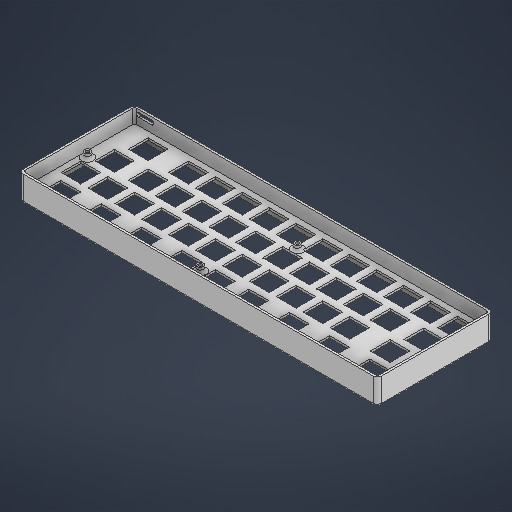
# Autodesk Inventor part: Top
Saved by Autodesk Inventor 2026 (Build 300175050, 175E)
## iProperties
Created: 2025-06-14
Part Number: Top
Material: Generisch
Document SubType Name: Modeling
Designer: nikla
Density: 1 g/cm^3
Appearance: Vorgabe
Author: nikla
Autodesk Inventor part; units mm, degrees
ref_plane "YZ Plane" through (0, 0, 0) normal (1, 0, 0) x (0, 1, 0)
ref_plane "XZ Plane" through (0, 0, 0) normal (0, 1, 0) x (-1, 0, 0)
ref_plane "XY Plane" through (0, 0, 0) normal (0, 0, 1) x (1, 0, 0)
sketch "Skizze1" plane through (0, 0, 0) normal (0, 0, 1) x (1, 0, 0)
  arc A0 (-233.4346, 67.6971) -> (-234.4346, 66.6971) centre (-233.4346, 66.6971) ccw projected
  line L0 (14.5654, 67.6971) -> (-233.4346, 67.6971) projected
  arc A1 (15.5654, 66.6971) -> (14.5654, 67.6971) centre (14.5654, 66.6971) ccw projected
  line L1 (15.5654, -9.3029) -> (15.5654, 66.6971) projected
  arc A2 (14.5654, -10.3029) -> (15.5654, -9.3029) centre (14.5654, -9.3029) ccw projected
  line L2 (-233.4346, -10.3029) -> (14.5654, -10.3029) projected
  arc A3 (-234.4346, -9.3029) -> (-233.4346, -10.3029) centre (-233.4346, -9.3029) ccw projected
  line L3 (-234.4346, 66.6971) -> (-234.4346, -9.3029) projected
  circle A4 centre (11.9054, -6.6429) radius 1.6 projected
  circle A5 centre (5.0729, 0.0071) radius 0.875 projected
  circle A6 centre (-0.0071, 0.0071) radius 2 projected
  circle A7 centre (-5.0871, 0.0071) radius 0.875 projected
  circle A8 centre (-23.5021, 0.0071) radius 0.875 projected
  circle A9 centre (-28.5821, 0.0071) radius 2 projected
  circle A10 centre (-33.6621, 0.0071) radius 0.875 projected
  circle A11 centre (3.8029, 2.5471) radius 0.75 projected
  circle A12 centre (-2.5471, 5.0871) radius 0.75 projected
  circle A13 centre (-24.7721, 2.5471) radius 0.75 projected
  circle A14 centre (-31.1221, 5.0871) radius 0.75 projected
  circle A15 centre (-52.0771, 0.0071) radius 0.875 projected
  circle A16 centre (-57.1571, 0.0071) radius 2 projected
  circle A17 centre (-62.2371, 0.0071) radius 0.875 projected
  circle A18 centre (-80.6521, 0.0071) radius 0.875 projected
  circle A19 centre (-85.7321, 0.0071) radius 2 projected
  circle A20 centre (-90.8121, 0.0071) radius 0.875 projected
  circle A21 centre (-104.4646, 0.0071) radius 0.875 projected
  circle A22 centre (-53.3471, 2.5471) radius 0.75 projected
  circle A23 centre (-59.6971, 5.0871) radius 0.75 projected
  circle A24 centre (-81.9221, 2.5471) radius 0.75 projected
  circle A25 centre (-88.2721, 5.0871) radius 0.75 projected
  circle A26 centre (-105.7346, 2.5471) radius 0.75 projected
  circle A27 centre (0.3104, 19.0571) radius 0.875 projected
  circle A28 centre (-0.9596, 21.5971) radius 0.75 projected
  circle A29 centre (-4.7696, 19.0571) radius 2 projected
  circle A30 centre (-9.8496, 19.0571) radius 0.875 projected
  circle A31 centre (-7.3096, 24.1371) radius 0.75 projected
  circle A32 centre (-28.2646, 19.0571) radius 0.875 projected
  circle A33 centre (-29.5346, 21.5971) radius 0.75 projected
  circle A34 centre (-33.3446, 19.0571) radius 2 projected
  circle A35 centre (-38.4246, 19.0571) radius 0.875 projected
  circle A36 centre (-47.3146, 19.0571) radius 0.875 projected
  circle A37 centre (-35.8846, 24.1371) radius 0.75 projected
  circle A38 centre (-52.3946, 19.0571) radius 2 projected
  circle A39 centre (-57.4746, 19.0571) radius 0.875 projected
  circle A40 centre (-48.5846, 21.5971) radius 0.75 projected
  circle A41 centre (-66.3646, 19.0571) radius 0.875 projected
  circle A42 centre (-71.4446, 19.0571) radius 2 projected
  circle A43 centre (-76.5246, 19.0571) radius 0.875 projected
  circle A44 centre (-67.6346, 21.5971) radius 0.75 projected
  circle A45 centre (-54.9346, 24.1371) radius 0.75 projected
  circle A46 centre (-73.9846, 24.1371) radius 0.75 projected
  circle A47 centre (-85.4146, 19.0571) radius 0.875 projected
  circle A48 centre (-90.4946, 19.0571) radius 2 projected
  circle A49 centre (-86.6846, 21.5971) radius 0.75 projected
  circle A50 centre (-95.5746, 19.0571) radius 0.875 projected
  circle A51 centre (-104.4646, 19.0571) radius 0.875 projected
  circle A52 centre (-105.7346, 21.5971) radius 0.75 projected
  circle A53 centre (-93.0346, 24.1371) radius 0.75 projected
  circle A54 centre (-109.5446, 0.0071) radius 2 projected
  circle A55 centre (-114.6246, 0.0071) radius 0.875 projected
  circle A56 centre (-128.2771, 0.0071) radius 0.875 projected
  circle A57 centre (-133.3571, 0.0071) radius 2 projected
  circle A58 centre (-138.4371, 0.0071) radius 0.875 projected
  circle A59 centre (-156.8521, 0.0071) radius 0.875 projected
  circle A60 centre (-161.9321, 0.0071) radius 2 projected
  circle A61 centre (-167.0121, 0.0071) radius 0.875 projected
  circle A62 centre (-121.1946, 0.9571) radius 1.6 projected
  circle A63 centre (-112.0846, 5.0871) radius 0.75 projected
  circle A64 centre (-129.5471, 2.5471) radius 0.75 projected
  circle A65 centre (-135.8971, 5.0871) radius 0.75 projected
  circle A66 centre (-158.1221, 2.5471) radius 0.75 projected
  circle A67 centre (-164.4721, 5.0871) radius 0.75 projected
  circle A68 centre (-185.4271, 0.0071) radius 0.875 projected
  circle A69 centre (-190.5071, 0.0071) radius 2 projected
  circle A70 centre (-195.5871, 0.0071) radius 0.875 projected
  circle A71 centre (-230.6946, -6.6429) radius 1.6 projected
  circle A72 centre (-214.0021, 0.0071) radius 0.875 projected
  circle A73 centre (-219.0821, 0.0071) radius 2 projected
  circle A74 centre (-224.1621, 0.0071) radius 0.875 projected
  circle A75 centre (-186.6971, 2.5471) radius 0.75 projected
  circle A76 centre (-193.0471, 5.0871) radius 0.75 projected
  circle A77 centre (-215.2721, 2.5471) radius 0.75 projected
  circle A78 centre (-221.6221, 5.0871) radius 0.75 projected
  circle A79 centre (-109.5446, 19.0571) radius 2 projected
  circle A80 centre (-114.6246, 19.0571) radius 0.875 projected
  circle A81 centre (-123.5146, 19.0571) radius 0.875 projected
  circle A82 centre (-128.5946, 19.0571) radius 2 projected
  circle A83 centre (-133.6746, 19.0571) radius 0.875 projected
  circle A84 centre (-124.7846, 21.5971) radius 0.75 projected
  circle A85 centre (-112.0846, 24.1371) radius 0.75 projected
  circle A86 centre (-131.1346, 24.1371) radius 0.75 projected
  circle A87 centre (-142.5646, 19.0571) radius 0.875 projected
  circle A88 centre (-147.6446, 19.0571) radius 2 projected
  circle A89 centre (-152.7246, 19.0571) radius 0.875 projected
  circle A90 centre (-143.8346, 21.5971) radius 0.75 projected
  circle A91 centre (-161.6146, 19.0571) radius 0.875 projected
  circle A92 centre (-166.6946, 19.0571) radius 2 projected
  circle A93 centre (-162.8846, 21.5971) radius 0.75 projected
  circle A94 centre (-150.1846, 24.1371) radius 0.75 projected
  circle A95 centre (-169.2346, 24.1371) radius 0.75 projected
  circle A96 centre (-171.7746, 19.0571) radius 0.875 projected
  circle A97 centre (-180.6646, 19.0571) radius 0.875 projected
  circle A98 centre (-185.7446, 19.0571) radius 2 projected
  circle A99 centre (-181.9346, 21.5971) radius 0.75 projected
  circle A100 centre (-190.8246, 19.0571) radius 0.875 projected
  circle A101 centre (-199.7146, 19.0571) radius 0.875 projected
  circle A102 centre (-200.9846, 21.5971) radius 0.75 projected
  circle A103 centre (-188.2846, 24.1371) radius 0.75 projected
  circle A104 centre (-204.7946, 19.0571) radius 2 projected
  circle A105 centre (-209.8746, 19.0571) radius 0.875 projected
  circle A106 centre (-218.7646, 19.0571) radius 0.875 projected
  circle A107 centre (-223.8446, 19.0571) radius 2 projected
  circle A108 centre (-228.9246, 19.0571) radius 0.875 projected
  circle A109 centre (-220.0346, 21.5971) radius 0.75 projected
  circle A110 centre (-207.3346, 24.1371) radius 0.75 projected
  circle A111 centre (-226.3846, 24.1371) radius 0.75 projected
  circle A112 centre (5.0729, 38.1071) radius 0.875 projected
  circle A113 centre (-0.0071, 38.1071) radius 2 projected
  circle A114 centre (3.8029, 40.6471) radius 0.75 projected
  circle A115 centre (-5.0871, 38.1071) radius 0.875 projected
  circle A116 centre (-2.5471, 43.1871) radius 0.75 projected
  circle A117 centre (-18.7396, 38.1071) radius 0.875 projected
  circle A118 centre (-23.8196, 38.1071) radius 2 projected
  circle A119 centre (-28.8996, 38.1071) radius 0.875 projected
  circle A120 centre (-20.0096, 40.6471) radius 0.75 projected
  circle A121 centre (-37.7896, 38.1071) radius 0.875 projected
  circle A122 centre (-42.8696, 38.1071) radius 2 projected
  circle A123 centre (-39.0596, 40.6471) radius 0.75 projected
  circle A124 centre (-26.3596, 43.1871) radius 0.75 projected
  circle A125 centre (-45.4096, 43.1871) radius 0.75 projected
  circle A126 centre (-47.9496, 38.1071) radius 0.875 projected
  circle A127 centre (-56.8396, 38.1071) radius 0.875 projected
  circle A128 centre (-61.9196, 38.1071) radius 2 projected
  circle A129 centre (-58.1096, 40.6471) radius 0.75 projected
  circle A130 centre (-66.9996, 38.1071) radius 0.875 projected
  circle A131 centre (-75.8896, 38.1071) radius 0.875 projected
  circle A132 centre (-77.1596, 40.6471) radius 0.75 projected
  circle A133 centre (-64.4596, 43.1871) radius 0.75 projected
  circle A134 centre (-80.9696, 38.1071) radius 2 projected
  circle A135 centre (-86.0496, 38.1071) radius 0.875 projected
  circle A136 centre (-94.9396, 38.1071) radius 0.875 projected
  circle A137 centre (-100.0196, 38.1071) radius 2 projected
  circle A138 centre (-105.0996, 38.1071) radius 0.875 projected
  circle A139 centre (-96.2096, 40.6471) radius 0.75 projected
  circle A140 centre (-83.5096, 43.1871) radius 0.75 projected
  circle A141 centre (-102.5596, 43.1871) radius 0.75 projected
  circle A142 centre (12.1054, 46.6571) radius 1.6 projected
  circle A143 centre (9.8354, 57.1571) radius 0.875 projected
  circle A144 centre (4.7554, 57.1571) radius 2 projected
  circle A145 centre (-0.3246, 57.1571) radius 0.875 projected
  circle A146 centre (-9.2146, 57.1571) radius 0.875 projected
  circle A147 centre (-14.2946, 57.1571) radius 2 projected
  circle A148 centre (8.5654, 59.6971) radius 0.75 projected
  circle A149 centre (2.2154, 62.2371) radius 0.75 projected
  circle A150 centre (-10.4846, 59.6971) radius 0.75 projected
  circle A151 centre (-16.8346, 62.2371) radius 0.75 projected
  circle A152 centre (-19.3746, 57.1571) radius 0.875 projected
  circle A153 centre (-28.2646, 57.1571) radius 0.875 projected
  circle A154 centre (-33.3446, 57.1571) radius 2 projected
  circle A155 centre (-38.4246, 57.1571) radius 0.875 projected
  circle A156 centre (-47.3146, 57.1571) radius 0.875 projected
  circle A157 centre (-29.5346, 59.6971) radius 0.75 projected
  circle A158 centre (-35.8846, 62.2371) radius 0.75 projected
  circle A159 centre (-100.1946, 48.7571) radius 1.6 projected
  circle A160 centre (-52.3946, 57.1571) radius 2 projected
  circle A161 centre (-57.4746, 57.1571) radius 0.875 projected
  circle A162 centre (-66.3646, 57.1571) radius 0.875 projected
  circle A163 centre (-71.4446, 57.1571) radius 2 projected
  circle A164 centre (-76.5246, 57.1571) radius 0.875 projected
  circle A165 centre (-48.5846, 59.6971) radius 0.75 projected
  circle A166 centre (-54.9346, 62.2371) radius 0.75 projected
  circle A167 centre (-67.6346, 59.6971) radius 0.75 projected
  circle A168 centre (-73.9846, 62.2371) radius 0.75 projected
  circle A169 centre (-85.4146, 57.1571) radius 0.875 projected
  circle A170 centre (-90.4946, 57.1571) radius 2 projected
  circle A171 centre (-95.5746, 57.1571) radius 0.875 projected
  circle A172 centre (-104.4646, 57.1571) radius 0.875 projected
  circle A173 centre (-86.6846, 59.6971) radius 0.75 projected
  circle A174 centre (-93.0346, 62.2371) radius 0.75 projected
  circle A175 centre (-105.7346, 59.6971) radius 0.75 projected
  circle A176 centre (-113.9896, 38.1071) radius 0.875 projected
  circle A177 centre (-119.0696, 38.1071) radius 2 projected
  circle A178 centre (-124.1496, 38.1071) radius 0.875 projected
  circle A179 centre (-115.2596, 40.6471) radius 0.75 projected
  circle A180 centre (-133.0396, 38.1071) radius 0.875 projected
  circle A181 centre (-138.1196, 38.1071) radius 2 projected
  circle A182 centre (-134.3096, 40.6471) radius 0.75 projected
  circle A183 centre (-121.6096, 43.1871) radius 0.75 projected
  circle A184 centre (-143.1996, 38.1071) radius 0.875 projected
  circle A185 centre (-152.0896, 38.1071) radius 0.875 projected
  circle A186 centre (-153.3596, 40.6471) radius 0.75 projected
  circle A187 centre (-157.1696, 38.1071) radius 2 projected
  circle A188 centre (-162.2496, 38.1071) radius 0.875 projected
  circle A189 centre (-140.6596, 43.1871) radius 0.75 projected
  circle A190 centre (-159.7096, 43.1871) radius 0.75 projected
  circle A191 centre (-230.7946, 30.6571) radius 1.6 projected
  circle A192 centre (-171.1396, 38.1071) radius 0.875 projected
  circle A193 centre (-176.2196, 38.1071) radius 2 projected
  circle A194 centre (-181.2996, 38.1071) radius 0.875 projected
  circle A195 centre (-172.4096, 40.6471) radius 0.75 projected
  circle A196 centre (-190.1896, 38.1071) radius 0.875 projected
  circle A197 centre (-195.2696, 38.1071) radius 2 projected
  circle A198 centre (-200.3496, 38.1071) radius 0.875 projected
  circle A199 centre (-191.4596, 40.6471) radius 0.75 projected
  circle A200 centre (-178.7596, 43.1871) radius 0.75 projected
  circle A201 centre (-197.8096, 43.1871) radius 0.75 projected
  circle A202 centre (-214.0021, 38.1071) radius 0.875 projected
  circle A203 centre (-215.2721, 40.6471) radius 0.75 projected
  circle A204 centre (-219.0821, 38.1071) radius 2 projected
  circle A205 centre (-224.1621, 38.1071) radius 0.875 projected
  circle A206 centre (-221.6221, 43.1871) radius 0.75 projected
  circle A207 centre (-109.5446, 57.1571) radius 2 projected
  circle A208 centre (-114.6246, 57.1571) radius 0.875 projected
  circle A209 centre (-123.5146, 57.1571) radius 0.875 projected
  circle A210 centre (-128.5946, 57.1571) radius 2 projected
  circle A211 centre (-133.6746, 57.1571) radius 0.875 projected
  circle A212 centre (-112.0846, 62.2371) radius 0.75 projected
  circle A213 centre (-124.7846, 59.6971) radius 0.75 projected
  circle A214 centre (-131.1346, 62.2371) radius 0.75 projected
  circle A215 centre (-142.5646, 57.1571) radius 0.875 projected
  circle A216 centre (-147.6446, 57.1571) radius 2 projected
  circle A217 centre (-152.7246, 57.1571) radius 0.875 projected
  circle A218 centre (-161.6146, 57.1571) radius 0.875 projected
  circle A219 centre (-166.6946, 57.1571) radius 2 projected
  circle A220 centre (-143.8346, 59.6971) radius 0.75 projected
  circle A221 centre (-150.1846, 62.2371) radius 0.75 projected
  circle A222 centre (-162.8846, 59.6971) radius 0.75 projected
  circle A223 centre (-169.2346, 62.2371) radius 0.75 projected
  circle A224 centre (-171.7746, 57.1571) radius 0.875 projected
  circle A225 centre (-180.6646, 57.1571) radius 0.875 projected
  circle A226 centre (-185.7446, 57.1571) radius 2 projected
  circle A227 centre (-190.8246, 57.1571) radius 0.875 projected
  circle A228 centre (-176.2946, 60.4571) radius 1.6 projected
  circle A229 centre (-181.9346, 59.6971) radius 0.75 projected
  circle A230 centre (-188.2846, 62.2371) radius 0.75 projected
  circle A231 centre (-209.2396, 57.1571) radius 0.875 projected
  circle A232 centre (-214.3196, 57.1571) radius 2 projected
  circle A233 centre (-219.3996, 57.1571) radius 0.875 projected
  arc A234 (-223.3846, 58.8771) -> (-222.7846, 58.8771) centre (-223.0846, 58.8771) ccw projected
  line L4 (-222.7846, 58.8771) -> (-222.7846, 59.9771) projected
  arc A235 (-222.7846, 59.9771) -> (-223.3846, 59.9771) centre (-223.0846, 59.9771) ccw projected
  line L5 (-223.3846, 59.9771) -> (-223.3846, 58.8771) projected
  arc A236 (-232.0246, 58.8771) -> (-231.4246, 58.8771) centre (-231.7246, 58.8771) ccw projected
  line L6 (-231.4246, 58.8771) -> (-231.4246, 59.9771) projected
  arc A237 (-231.4246, 59.9771) -> (-232.0246, 59.9771) centre (-231.7246, 59.9771) ccw projected
  line L7 (-232.0246, 59.9771) -> (-232.0246, 58.8771) projected
  circle A238 centre (-210.5096, 59.6971) radius 0.75 projected
  circle A239 centre (-216.8596, 62.2371) radius 0.75 projected
  circle A240 centre (-224.5146, 59.9571) radius 0.325 projected
  circle A241 centre (-230.2946, 59.9571) radius 0.325 projected
  arc A242 (-223.3846, 63.3071) -> (-222.7846, 63.3071) centre (-223.0846, 63.3071) ccw projected
  line L8 (-222.7846, 63.3071) -> (-222.7846, 63.9071) projected
  arc A243 (-222.7846, 63.9071) -> (-223.3846, 63.9071) centre (-223.0846, 63.9071) ccw projected
  line L9 (-223.3846, 63.9071) -> (-223.3846, 63.3071) projected
  arc A244 (-232.0246, 63.3071) -> (-231.4246, 63.3071) centre (-231.7246, 63.3071) ccw projected
  line L10 (-231.4246, 63.3071) -> (-231.4246, 63.9071) projected
  arc A245 (-231.4246, 63.9071) -> (-232.0246, 63.9071) centre (-231.7246, 63.9071) ccw projected
  line L11 (-232.0246, 63.9071) -> (-232.0246, 63.3071) projected
  line L12 (11.7554, 50.1571) -> (-2.2446, 50.1571)
  line L13 (-2.2446, 50.1571) -> (-2.2446, 64.1571)
  line L14 (-2.2446, 64.1571) -> (11.7554, 64.1571)
  line L15 (11.7554, 64.1571) -> (11.7554, 50.1571)
  line L16 (11.7554, 50.1571) -> (-2.2446, 64.1571) construction
  line L17 (-2.2446, 50.1571) -> (11.7554, 64.1571) construction
  line L18 (-21.2946, 50.1571) -> (-7.2946, 50.1571)
  line L19 (-7.2946, 50.1571) -> (-7.2946, 64.1571)
  line L20 (-7.2946, 64.1571) -> (-21.2946, 64.1571)
  line L21 (-21.2946, 64.1571) -> (-21.2946, 50.1571)
  line L22 (-21.2946, 50.1571) -> (-7.2946, 64.1571) construction
  line L23 (-7.2946, 50.1571) -> (-21.2946, 64.1571) construction
  line L24 (-7.0071, 31.1071) -> (6.9929, 31.1071)
  line L25 (6.9929, 31.1071) -> (6.9929, 45.1071)
  line L26 (6.9929, 45.1071) -> (-7.0071, 45.1071)
  line L27 (-7.0071, 45.1071) -> (-7.0071, 31.1071)
  line L28 (-7.0071, 31.1071) -> (6.9929, 45.1071) construction
  line L29 (6.9929, 31.1071) -> (-7.0071, 45.1071) construction
  line L30 (-30.8196, 31.1071) -> (-16.8196, 31.1071)
  line L31 (-16.8196, 31.1071) -> (-16.8196, 45.1071)
  line L32 (-16.8196, 45.1071) -> (-30.8196, 45.1071)
  line L33 (-30.8196, 45.1071) -> (-30.8196, 31.1071)
  line L34 (-30.8196, 31.1071) -> (-16.8196, 45.1071) construction
  line L35 (-16.8196, 31.1071) -> (-30.8196, 45.1071) construction
  line L36 (-40.3446, 50.1571) -> (-26.3446, 50.1571)
  line L37 (-26.3446, 50.1571) -> (-26.3446, 64.1571)
  line L38 (-26.3446, 64.1571) -> (-40.3446, 64.1571)
  line L39 (-40.3446, 64.1571) -> (-40.3446, 50.1571)
  line L40 (-40.3446, 50.1571) -> (-26.3446, 64.1571) construction
  line L41 (-26.3446, 50.1571) -> (-40.3446, 64.1571) construction
  line L42 (-35.8696, 31.1071) -> (-49.8696, 31.1071)
  line L43 (-49.8696, 31.1071) -> (-49.8696, 45.1071)
  line L44 (-49.8696, 45.1071) -> (-35.8696, 45.1071)
  line L45 (-35.8696, 45.1071) -> (-35.8696, 31.1071)
  line L46 (-35.8696, 31.1071) -> (-49.8696, 45.1071) construction
  line L47 (-49.8696, 31.1071) -> (-35.8696, 45.1071) construction
  line L48 (-45.3946, 50.1571) -> (-59.3946, 50.1571)
  line L49 (-59.3946, 50.1571) -> (-59.3946, 64.1571)
  line L50 (-59.3946, 64.1571) -> (-45.3946, 64.1571)
  line L51 (-45.3946, 64.1571) -> (-45.3946, 50.1571)
  line L52 (-45.3946, 50.1571) -> (-59.3946, 64.1571) construction
  line L53 (-59.3946, 50.1571) -> (-45.3946, 64.1571) construction
  line L54 (-54.9196, 31.1071) -> (-68.9196, 31.1071)
  line L55 (-68.9196, 31.1071) -> (-68.9196, 45.1071)
  line L56 (-68.9196, 45.1071) -> (-54.9196, 45.1071)
  line L57 (-54.9196, 45.1071) -> (-54.9196, 31.1071)
  line L58 (-54.9196, 31.1071) -> (-68.9196, 45.1071) construction
  line L59 (-68.9196, 31.1071) -> (-54.9196, 45.1071) construction
  line L60 (-78.4446, 50.1571) -> (-64.4446, 50.1571)
  line L61 (-64.4446, 50.1571) -> (-64.4446, 64.1571)
  line L62 (-64.4446, 64.1571) -> (-78.4446, 64.1571)
  line L63 (-78.4446, 64.1571) -> (-78.4446, 50.1571)
  line L64 (-78.4446, 50.1571) -> (-64.4446, 64.1571) construction
  line L65 (-64.4446, 50.1571) -> (-78.4446, 64.1571) construction
  line L66 (-87.9696, 31.1071) -> (-73.9696, 31.1071)
  line L67 (-73.9696, 31.1071) -> (-73.9696, 45.1071)
  line L68 (-73.9696, 45.1071) -> (-87.9696, 45.1071)
  line L69 (-87.9696, 45.1071) -> (-87.9696, 31.1071)
  line L70 (-87.9696, 31.1071) -> (-73.9696, 45.1071) construction
  line L71 (-73.9696, 31.1071) -> (-87.9696, 45.1071) construction
  line L72 (-83.4946, 64.1571) -> (-97.4946, 64.1571)
  line L73 (-97.4946, 64.1571) -> (-97.4946, 50.1571)
  line L74 (-97.4946, 50.1571) -> (-83.4946, 50.1571)
  line L75 (-83.4946, 50.1571) -> (-83.4946, 64.1571)
  line L76 (-83.4946, 64.1571) -> (-97.4946, 50.1571) construction
  line L77 (-97.4946, 64.1571) -> (-83.4946, 50.1571) construction
  line L78 (-93.0196, 31.1071) -> (-107.0196, 31.1071)
  line L79 (-107.0196, 31.1071) -> (-107.0196, 45.1071)
  line L80 (-107.0196, 45.1071) -> (-93.0196, 45.1071)
  line L81 (-93.0196, 45.1071) -> (-93.0196, 31.1071)
  line L82 (-93.0196, 31.1071) -> (-107.0196, 45.1071) construction
  line L83 (-107.0196, 31.1071) -> (-93.0196, 45.1071) construction
  line L84 (-102.5446, 50.1571) -> (-116.5446, 50.1571)
  line L85 (-116.5446, 50.1571) -> (-116.5446, 64.1571)
  line L86 (-116.5446, 64.1571) -> (-102.5446, 64.1571)
  line L87 (-102.5446, 64.1571) -> (-102.5446, 50.1571)
  line L88 (-102.5446, 50.1571) -> (-116.5446, 64.1571) construction
  line L89 (-116.5446, 50.1571) -> (-102.5446, 64.1571) construction
  line L90 (-126.0696, 31.1071) -> (-112.0696, 31.1071)
  line L91 (-112.0696, 31.1071) -> (-112.0696, 45.1071)
  line L92 (-112.0696, 45.1071) -> (-126.0696, 45.1071)
  line L93 (-126.0696, 45.1071) -> (-126.0696, 31.1071)
  line L94 (-126.0696, 31.1071) -> (-112.0696, 45.1071) construction
  line L95 (-112.0696, 31.1071) -> (-126.0696, 45.1071) construction
  line L96 (-121.5946, 64.1571) -> (-135.5946, 64.1571)
  line L97 (-135.5946, 64.1571) -> (-135.5946, 50.1571)
  line L98 (-135.5946, 50.1571) -> (-121.5946, 50.1571)
  line L99 (-121.5946, 50.1571) -> (-121.5946, 64.1571)
  line L100 (-121.5946, 64.1571) -> (-135.5946, 50.1571) construction
  line L101 (-135.5946, 64.1571) -> (-121.5946, 50.1571) construction
  line L102 (-131.1196, 31.1071) -> (-145.1196, 31.1071)
  line L103 (-145.1196, 31.1071) -> (-145.1196, 45.1071)
  line L104 (-145.1196, 45.1071) -> (-131.1196, 45.1071)
  line L105 (-131.1196, 45.1071) -> (-131.1196, 31.1071)
  line L106 (-131.1196, 31.1071) -> (-145.1196, 45.1071) construction
  line L107 (-145.1196, 31.1071) -> (-131.1196, 45.1071) construction
  line L108 (-154.6446, 50.1571) -> (-140.6446, 50.1571)
  line L109 (-140.6446, 50.1571) -> (-140.6446, 64.1571)
  line L110 (-140.6446, 64.1571) -> (-154.6446, 64.1571)
  line L111 (-154.6446, 64.1571) -> (-154.6446, 50.1571)
  line L112 (-154.6446, 50.1571) -> (-140.6446, 64.1571) construction
  line L113 (-140.6446, 50.1571) -> (-154.6446, 64.1571) construction
  line L114 (-164.1696, 45.1071) -> (-150.1696, 45.1071)
  line L115 (-150.1696, 45.1071) -> (-150.1696, 31.1071)
  line L116 (-150.1696, 31.1071) -> (-164.1696, 31.1071)
  line L117 (-164.1696, 31.1071) -> (-164.1696, 45.1071)
  line L118 (-164.1696, 45.1071) -> (-150.1696, 31.1071) construction
  line L119 (-150.1696, 45.1071) -> (-164.1696, 31.1071) construction
  line L120 (-159.6946, 50.1571) -> (-173.6946, 50.1571)
  line L121 (-173.6946, 50.1571) -> (-173.6946, 64.1571)
  line L122 (-173.6946, 64.1571) -> (-159.6946, 64.1571)
  line L123 (-159.6946, 64.1571) -> (-159.6946, 50.1571)
  line L124 (-159.6946, 50.1571) -> (-173.6946, 64.1571) construction
  line L125 (-173.6946, 50.1571) -> (-159.6946, 64.1571) construction
  line L126 (-183.2196, 45.1071) -> (-169.2196, 45.1071)
  line L127 (-169.2196, 45.1071) -> (-169.2196, 31.1071)
  line L128 (-169.2196, 31.1071) -> (-183.2196, 31.1071)
  line L129 (-183.2196, 31.1071) -> (-183.2196, 45.1071)
  line L130 (-183.2196, 45.1071) -> (-169.2196, 31.1071) construction
  line L131 (-169.2196, 45.1071) -> (-183.2196, 31.1071) construction
  line L132 (-192.7446, 64.1571) -> (-178.7446, 64.1571)
  line L133 (-178.7446, 64.1571) -> (-178.7446, 50.1571)
  line L134 (-178.7446, 50.1571) -> (-192.7446, 50.1571)
  line L135 (-192.7446, 50.1571) -> (-192.7446, 64.1571)
  line L136 (-192.7446, 64.1571) -> (-178.7446, 50.1571) construction
  line L137 (-178.7446, 64.1571) -> (-192.7446, 50.1571) construction
  line L138 (-188.2696, 31.1071) -> (-202.2696, 31.1071)
  line L139 (-202.2696, 31.1071) -> (-202.2696, 45.1071)
  line L140 (-202.2696, 45.1071) -> (-188.2696, 45.1071)
  line L141 (-188.2696, 45.1071) -> (-188.2696, 31.1071)
  line L142 (-188.2696, 31.1071) -> (-202.2696, 45.1071) construction
  line L143 (-202.2696, 31.1071) -> (-188.2696, 45.1071) construction
  line L144 (-207.3196, 64.1571) -> (-221.3196, 64.1571)
  line L145 (-221.3196, 64.1571) -> (-221.3196, 50.1571)
  line L146 (-221.3196, 50.1571) -> (-207.3196, 50.1571)
  line L147 (-207.3196, 50.1571) -> (-207.3196, 64.1571)
  line L148 (-207.3196, 64.1571) -> (-221.3196, 50.1571) construction
  line L149 (-221.3196, 64.1571) -> (-207.3196, 50.1571) construction
  line L150 (-212.0821, 31.1071) -> (-226.0821, 31.1071)
  line L151 (-226.0821, 31.1071) -> (-226.0821, 45.1071)
  line L152 (-226.0821, 45.1071) -> (-212.0821, 45.1071)
  line L153 (-212.0821, 45.1071) -> (-212.0821, 31.1071)
  line L154 (-212.0821, 31.1071) -> (-226.0821, 45.1071) construction
  line L155 (-226.0821, 31.1071) -> (-212.0821, 45.1071) construction
  line L156 (-216.8446, 26.0571) -> (-230.8446, 26.0571)
  line L157 (-230.8446, 26.0571) -> (-230.8446, 12.0571)
  line L158 (-230.8446, 12.0571) -> (-216.8446, 12.0571)
  line L159 (-216.8446, 12.0571) -> (-216.8446, 26.0571)
  line L160 (-216.8446, 26.0571) -> (-230.8446, 12.0571) construction
  line L161 (-230.8446, 26.0571) -> (-216.8446, 12.0571) construction
  line L162 (-212.0821, 7.0071) -> (-226.0821, 7.0071)
  line L163 (-226.0821, 7.0071) -> (-226.0821, -6.9929)
  line L164 (-226.0821, -6.9929) -> (-212.0821, -6.9929)
  line L165 (-212.0821, -6.9929) -> (-212.0821, 7.0071)
  line L166 (-212.0821, 7.0071) -> (-226.0821, -6.9929) construction
  line L167 (-226.0821, 7.0071) -> (-212.0821, -6.9929) construction
  line L168 (-197.7946, 12.0571) -> (-211.7946, 12.0571)
  line L169 (-211.7946, 12.0571) -> (-211.7946, 26.0571)
  line L170 (-211.7946, 26.0571) -> (-197.7946, 26.0571)
  line L171 (-197.7946, 26.0571) -> (-197.7946, 12.0571)
  line L172 (-197.7946, 12.0571) -> (-211.7946, 26.0571) construction
  line L173 (-211.7946, 12.0571) -> (-197.7946, 26.0571) construction
  line L174 (-192.7446, 26.0571) -> (-178.7446, 26.0571)
  line L175 (-178.7446, 26.0571) -> (-178.7446, 12.0571)
  line L176 (-178.7446, 12.0571) -> (-192.7446, 12.0571)
  line L177 (-192.7446, 12.0571) -> (-192.7446, 26.0571)
  line L178 (-192.7446, 26.0571) -> (-178.7446, 12.0571) construction
  line L179 (-178.7446, 26.0571) -> (-192.7446, 12.0571) construction
  line L180 (-183.5071, -6.9929) -> (-197.5071, -6.9929)
  line L181 (-197.5071, -6.9929) -> (-197.5071, 7.0071)
  line L182 (-197.5071, 7.0071) -> (-183.5071, 7.0071)
  line L183 (-183.5071, 7.0071) -> (-183.5071, -6.9929)
  line L184 (-183.5071, -6.9929) -> (-197.5071, 7.0071) construction
  line L185 (-197.5071, -6.9929) -> (-183.5071, 7.0071) construction
  line L186 (-173.6946, 26.0571) -> (-159.6946, 26.0571)
  line L187 (-159.6946, 26.0571) -> (-159.6946, 12.0571)
  line L188 (-159.6946, 12.0571) -> (-173.6946, 12.0571)
  line L189 (-173.6946, 12.0571) -> (-173.6946, 26.0571)
  line L190 (-173.6946, 26.0571) -> (-159.6946, 12.0571) construction
  line L191 (-159.6946, 26.0571) -> (-173.6946, 12.0571) construction
  line L192 (-154.6446, 26.0571) -> (-140.6446, 26.0571)
  line L193 (-140.6446, 26.0571) -> (-140.6446, 12.0571)
  line L194 (-140.6446, 12.0571) -> (-154.6446, 12.0571)
  line L195 (-154.6446, 12.0571) -> (-154.6446, 26.0571)
  line L196 (-154.6446, 26.0571) -> (-140.6446, 12.0571) construction
  line L197 (-140.6446, 26.0571) -> (-154.6446, 12.0571) construction
  line L198 (-168.9321, -6.9929) -> (-154.9321, -6.9929)
  line L199 (-154.9321, -6.9929) -> (-154.9321, 7.0071)
  line L200 (-154.9321, 7.0071) -> (-168.9321, 7.0071)
  line L201 (-168.9321, 7.0071) -> (-168.9321, -6.9929)
  line L202 (-168.9321, -6.9929) -> (-154.9321, 7.0071) construction
  line L203 (-154.9321, -6.9929) -> (-168.9321, 7.0071) construction
  line L204 (-126.3571, -6.9929) -> (-140.3571, -6.9929)
  line L205 (-140.3571, -6.9929) -> (-140.3571, 7.0071)
  line L206 (-140.3571, 7.0071) -> (-126.3571, 7.0071)
  line L207 (-126.3571, 7.0071) -> (-126.3571, -6.9929)
  line L208 (-126.3571, -6.9929) -> (-140.3571, 7.0071) construction
  line L209 (-140.3571, -6.9929) -> (-126.3571, 7.0071) construction
  line L210 (-121.5946, 26.0571) -> (-135.5946, 26.0571)
  line L211 (-135.5946, 26.0571) -> (-135.5946, 12.0571)
  line L212 (-135.5946, 12.0571) -> (-121.5946, 12.0571)
  line L213 (-121.5946, 12.0571) -> (-121.5946, 26.0571)
  line L214 (-121.5946, 26.0571) -> (-135.5946, 12.0571) construction
  line L215 (-135.5946, 26.0571) -> (-121.5946, 12.0571) construction
  line L216 (-102.5446, 26.0571) -> (-116.5446, 26.0571)
  line L217 (-116.5446, 26.0571) -> (-116.5446, 12.0571)
  line L218 (-116.5446, 12.0571) -> (-102.5446, 12.0571)
  line L219 (-102.5446, 12.0571) -> (-102.5446, 26.0571)
  line L220 (-102.5446, 26.0571) -> (-116.5446, 12.0571) construction
  line L221 (-116.5446, 26.0571) -> (-102.5446, 12.0571) construction
  line L222 (-102.5446, 7.0071) -> (-116.5446, 7.0071)
  line L223 (-116.5446, 7.0071) -> (-116.5446, -6.9929)
  line L224 (-116.5446, -6.9929) -> (-102.5446, -6.9929)
  line L225 (-102.5446, -6.9929) -> (-102.5446, 7.0071)
  line L226 (-102.5446, 7.0071) -> (-116.5446, -6.9929) construction
  line L227 (-116.5446, 7.0071) -> (-102.5446, -6.9929) construction
  line L228 (-83.4946, 26.0571) -> (-97.4946, 26.0571)
  line L229 (-97.4946, 26.0571) -> (-97.4946, 12.0571)
  line L230 (-97.4946, 12.0571) -> (-83.4946, 12.0571)
  line L231 (-83.4946, 12.0571) -> (-83.4946, 26.0571)
  line L232 (-83.4946, 26.0571) -> (-97.4946, 12.0571) construction
  line L233 (-97.4946, 26.0571) -> (-83.4946, 12.0571) construction
  line L234 (-78.7321, 7.0071) -> (-92.7321, 7.0071)
  line L235 (-92.7321, 7.0071) -> (-92.7321, -6.9929)
  line L236 (-92.7321, -6.9929) -> (-78.7321, -6.9929)
  line L237 (-78.7321, -6.9929) -> (-78.7321, 7.0071)
  line L238 (-78.7321, 7.0071) -> (-92.7321, -6.9929) construction
  line L239 (-92.7321, 7.0071) -> (-78.7321, -6.9929) construction
  line L240 (-64.1571, 7.0071) -> (-50.1571, 7.0071)
  line L241 (-50.1571, 7.0071) -> (-50.1571, -6.9929)
  line L242 (-50.1571, -6.9929) -> (-64.1571, -6.9929)
  line L243 (-64.1571, -6.9929) -> (-64.1571, 7.0071)
  line L244 (-64.1571, 7.0071) -> (-50.1571, -6.9929) construction
  line L245 (-50.1571, 7.0071) -> (-64.1571, -6.9929) construction
  line L246 (-64.4446, 26.0571) -> (-78.4446, 26.0571)
  line L247 (-78.4446, 26.0571) -> (-78.4446, 12.0571)
  line L248 (-78.4446, 12.0571) -> (-64.4446, 12.0571)
  line L249 (-64.4446, 12.0571) -> (-64.4446, 26.0571)
  line L250 (-64.4446, 26.0571) -> (-78.4446, 12.0571) construction
  line L251 (-78.4446, 26.0571) -> (-64.4446, 12.0571) construction
  line L252 (-45.3946, 26.0571) -> (-59.3946, 26.0571)
  line L253 (-59.3946, 26.0571) -> (-59.3946, 12.0571)
  line L254 (-59.3946, 12.0571) -> (-45.3946, 12.0571)
  line L255 (-45.3946, 12.0571) -> (-45.3946, 26.0571)
  line L256 (-45.3946, 26.0571) -> (-59.3946, 12.0571) construction
  line L257 (-59.3946, 26.0571) -> (-45.3946, 12.0571) construction
  line L258 (-40.3446, 12.0571) -> (-26.3446, 12.0571)
  line L259 (-26.3446, 12.0571) -> (-26.3446, 26.0571)
  line L260 (-26.3446, 26.0571) -> (-40.3446, 26.0571)
  line L261 (-40.3446, 26.0571) -> (-40.3446, 12.0571)
  line L262 (-40.3446, 12.0571) -> (-26.3446, 26.0571) construction
  line L263 (-26.3446, 12.0571) -> (-40.3446, 26.0571) construction
  line L264 (-35.5821, 7.0071) -> (-21.5821, 7.0071)
  line L265 (-21.5821, 7.0071) -> (-21.5821, -6.9929)
  line L266 (-21.5821, -6.9929) -> (-35.5821, -6.9929)
  line L267 (-35.5821, -6.9929) -> (-35.5821, 7.0071)
  line L268 (-35.5821, 7.0071) -> (-21.5821, -6.9929) construction
  line L269 (-21.5821, 7.0071) -> (-35.5821, -6.9929) construction
  line L270 (2.2304, 26.0571) -> (-11.7696, 26.0571)
  line L271 (-11.7696, 26.0571) -> (-11.7696, 12.0571)
  line L272 (-11.7696, 12.0571) -> (2.2304, 12.0571)
  line L273 (2.2304, 12.0571) -> (2.2304, 26.0571)
  line L274 (2.2304, 26.0571) -> (-11.7696, 12.0571) construction
  line L275 (-11.7696, 26.0571) -> (2.2304, 12.0571) construction
  line L276 (6.9929, -6.9929) -> (-7.0071, -6.9929)
  line L277 (-7.0071, -6.9929) -> (-7.0071, 7.0071)
  line L278 (-7.0071, 7.0071) -> (6.9929, 7.0071)
  line L279 (6.9929, 7.0071) -> (6.9929, -6.9929)
  line L280 (6.9929, -6.9929) -> (-7.0071, 7.0071) construction
  line L281 (-7.0071, -6.9929) -> (6.9929, 7.0071) construction
  arc A246 (-233.4346, 69.6971) -> (-236.4346, 66.6971) centre (-233.4346, 66.6971) ccw
  line L282 (-236.4346, 66.6971) -> (-236.4346, -9.3029)
  arc A247 (-236.4346, -9.3029) -> (-233.4346, -12.3029) centre (-233.4346, -9.3029) ccw
  line L283 (-233.4346, -12.3029) -> (14.5654, -12.3029)
  arc A248 (14.5654, -12.3029) -> (17.5654, -9.3029) centre (14.5654, -9.3029) ccw
  line L284 (17.5654, -9.3029) -> (17.5654, 66.6971)
  arc A249 (17.5654, 66.6971) -> (14.5654, 69.6971) centre (14.5654, 66.6971) ccw
  line L285 (14.5654, 69.6971) -> (-233.4346, 69.6971)
  arc A250 (16.0654, 66.6971) -> (14.5654, 68.1971) centre (14.5654, 66.6971) ccw
  line L286 (16.0654, 66.6971) -> (16.0654, -9.3029)
  arc A251 (14.5654, -10.8029) -> (16.0654, -9.3029) centre (14.5654, -9.3029) ccw
  line L287 (14.5654, -10.8029) -> (-233.4346, -10.8029)
  arc A252 (-234.9346, -9.3029) -> (-233.4346, -10.8029) centre (-233.4346, -9.3029) ccw
  line L288 (-234.9346, -9.3029) -> (-234.9346, 66.6971)
  arc A253 (-233.4346, 68.1971) -> (-234.9346, 66.6971) centre (-233.4346, 66.6971) ccw
  line L289 (-233.4346, 68.1971) -> (14.5654, 68.1971)
  point P0 (0, 0)
  dimension "d0" = 14
  dimension "d1" = 14
  dimension "d2" = 14
  dimension "d3" = 14
  dimension "d4" = 14
  dimension "d5" = 14
  dimension "d6" = 14
  dimension "d7" = 14
  dimension "d8" = 14
  dimension "d9" = 14
  dimension "d10" = 14
  dimension "d11" = 14
  dimension "d12" = 14
  dimension "d13" = 14
  dimension "d14" = 14
  dimension "d15" = 14
  dimension "d16" = 14
  dimension "d17" = 14
  dimension "d18" = 14
  dimension "d19" = 14
  dimension "d20" = 14
  dimension "d21" = 14
  dimension "d22" = 14
  dimension "d23" = 14
  dimension "d24" = 14
  dimension "d25" = 14
  dimension "d26" = 14
  dimension "d27" = 14
  dimension "d28" = 14
  dimension "d29" = 14
  dimension "d30" = 14
  dimension "d31" = 14
  dimension "d32" = 14
  dimension "d33" = 14
  dimension "d34" = 14
  dimension "d35" = 14
  dimension "d36" = 14
  dimension "d37" = 14
  dimension "d38" = 14
  dimension "d39" = 14
  dimension "d40" = 14
  dimension "d41" = 14
  dimension "d42" = 14
  dimension "d43" = 14
  dimension "d44" = 14
  dimension "d45" = 14
  dimension "d46" = 14
  dimension "d47" = 14
  dimension "d48" = 14
  dimension "d49" = 14
  dimension "d50" = 14
  dimension "d51" = 14
  dimension "d52" = 14
  dimension "d53" = 14
  dimension "d54" = 14
  dimension "d55" = 14
  dimension "d56" = 14
  dimension "d57" = 14
  dimension "d58" = 14
  dimension "d59" = 14
  dimension "d60" = 14
  dimension "d61" = 14
  dimension "d62" = 14
  dimension "d63" = 14
  constraints: 556 end point, 90 midpoint, 90 parallel, 45 horizontal, 45 perpendicular, 16 point on circle, 8 centre point, 14 other
  measures "d0" distance of L13.end L14.end
  measures "d1" distance of L12.end L13.end
  measures "d2" distance of L20.end L19.end
  measures "d3" distance of L19.end L18.end
  measures "d4" distance of L26.end L25.end
  measures "d5" distance of L25.end L24.end
  measures "d6" distance of L32.end L31.end
  measures "d7" distance of L31.end L30.end
  measures "d8" distance of L38.end L37.end
  measures "d9" distance of L37.end L36.end
  measures "d10" distance of L43.end L44.end
  measures "d11" distance of L42.end L43.end
  measures "d12" distance of L49.end L50.end
  measures "d13" distance of L48.end L49.end
  measures "d14" distance of L55.end L56.end
  measures "d15" distance of L54.end L55.end
  measures "d16" distance of L62.end L61.end
  measures "d17" distance of L61.end L60.end
  measures "d18" distance of L68.end L67.end
  measures "d19" distance of L67.end L66.end
  measures "d20" distance of L74.end L73.end
  measures "d21" distance of L73.end L72.end
  measures "d22" distance of L79.end L80.end
  measures "d23" distance of L78.end L79.end
  measures "d24" distance of L85.end L86.end
  measures "d25" distance of L84.end L85.end
  measures "d26" distance of L92.end L91.end
  measures "d27" distance of L91.end L90.end
  measures "d28" distance of L98.end L97.end
  measures "d29" distance of L97.end L96.end
  measures "d30" distance of L103.end L104.end
  measures "d31" distance of L102.end L103.end
  measures "d32" distance of L110.end L109.end
  measures "d33" distance of L109.end L108.end
  measures "d34" distance of L115.end L116.end
  measures "d35" distance of L114.end L115.end
  measures "d36" distance of L121.end L122.end
  measures "d37" distance of L120.end L121.end
  measures "d38" distance of L127.end L128.end
  measures "d39" distance of L126.end L127.end
  measures "d40" distance of L133.end L134.end
  measures "d41" distance of L132.end L133.end
  measures "d42" distance of L139.end L140.end
  measures "d43" distance of L138.end L139.end
  measures "d44" distance of L146.end L145.end
  measures "d45" distance of L145.end L144.end
  measures "d46" distance of L151.end L152.end
  measures "d47" distance of L150.end L151.end
  measures "d48" distance of L158.end L157.end
  measures "d49" distance of L157.end L156.end
  measures "d50" distance of L164.end L163.end
  measures "d51" distance of L163.end L162.end
  measures "d52" distance of L169.end L170.end
  measures "d53" distance of L168.end L169.end
  measures "d54" distance of L175.end L176.end
  measures "d55" distance of L174.end L175.end
  measures "d56" distance of L181.end L182.end
  measures "d57" distance of L180.end L181.end
  measures "d58" distance of L187.end L188.end
  measures "d59" distance of L186.end L187.end
  measures "d60" distance of L193.end L194.end
  measures "d61" distance of L192.end L193.end
  measures "d62" distance of L200.end L199.end
  measures "d63" distance of L199.end L198.end
extrude "Extrusion1" add sketch "Skizze1" along normal blind 1.5 contours L0 A1 L1 A2 L2 A3 L3 A0 | A4 | A62 | A71 | A142 | A159 | A191 | A228 | L5 A235 L4 A234 | L7 A237 L6 A236 | A240 | A241 | L9 A243 L8 A242 | L11 A245 L10 A244 | L285 A249 L284 A248 L283 A247 L282 A246 | L286 A251 L287 A252 L288 A253 L289 A250
sketch "Skizze2" plane through (0, 0, 1.5) normal (0, 0, 1) x (1, 0, 0)
  line L0 (-233.4346, -12.3029) -> (14.5654, -12.3029) projected
  arc A0 (14.5654, -12.3029) -> (17.5654, -9.3029) centre (14.5654, -9.3029) ccw projected
  line L1 (17.5654, -9.3029) -> (17.5654, 66.6971) projected
  arc A1 (17.5654, 66.6971) -> (14.5654, 69.6971) centre (14.5654, 66.6971) ccw projected
  line L2 (14.5654, 69.6971) -> (-233.4346, 69.6971) projected
  arc A2 (-233.4346, 69.6971) -> (-236.4346, 66.6971) centre (-233.4346, 66.6971) ccw projected
  line L3 (-236.4346, 66.6971) -> (-236.4346, -9.3029) projected
  arc A3 (-236.4346, -9.3029) -> (-233.4346, -12.3029) centre (-233.4346, -9.3029) ccw projected
  line L4 (14.5654, -10.8029) -> (-233.4346, -10.8029)
  arc A4 (-234.9346, -9.3029) -> (-233.4346, -10.8029) centre (-233.4346, -9.3029) ccw
  line L5 (-234.9346, -9.3029) -> (-234.9346, 66.6971)
  arc A5 (-233.4346, 68.1971) -> (-234.9346, 66.6971) centre (-233.4346, 66.6971) ccw
  line L6 (-233.4346, 68.1971) -> (14.5654, 68.1971)
  arc A6 (16.0654, 66.6971) -> (14.5654, 68.1971) centre (14.5654, 66.6971) ccw
  line L7 (16.0654, 66.6971) -> (16.0654, -9.3029)
  arc A7 (14.5654, -10.8029) -> (16.0654, -9.3029) centre (14.5654, -9.3029) ccw
  point P0 (0, 0)
  dimension "d94" = 1.5
  constraints: 8 end point, 8 point on circle, 4 centre point, 7 other
  measures "d94" distance between parallel lines of L0 L4
extrude "Extrusion2" add sketch "Skizze2" along normal blind 10
sketch "Skizze3" plane through (0, 0, 0) normal (0, 0, -1) x (-1, 0, 0)
  line L0 (-17.5654, -9.3029) -> (-17.5654, 66.6971) projected
  arc A0 (-17.5654, -9.3029) -> (-14.5654, -12.3029) centre (-14.5654, -9.3029) ccw projected
  line L1 (233.4346, -12.3029) -> (-14.5654, -12.3029) projected
  arc A1 (-14.5654, 69.6971) -> (-17.5654, 66.6971) centre (-14.5654, 66.6971) ccw projected
  line L2 (-14.5654, 69.6971) -> (233.4346, 69.6971) projected
  arc A2 (236.4346, 66.6971) -> (233.4346, 69.6971) centre (233.4346, 66.6971) ccw projected
  line L3 (236.4346, 66.6971) -> (236.4346, -9.3029) projected
  arc A3 (233.4346, -12.3029) -> (236.4346, -9.3029) centre (233.4346, -9.3029) ccw projected
  line L4 (234.4346, -9.3029) -> (234.4346, 66.6971)
  arc A4 (234.4346, 66.6971) -> (233.4346, 67.6971) centre (233.4346, 66.6971) ccw
  line L5 (233.4346, 67.6971) -> (-14.5654, 67.6971)
  arc A5 (-14.5654, 67.6971) -> (-15.5654, 66.6971) centre (-14.5654, 66.6971) ccw
  line L6 (-15.5654, 66.6971) -> (-15.5654, -9.3029)
  arc A6 (-15.5654, -9.3029) -> (-14.5654, -10.3029) centre (-14.5654, -9.3029) ccw
  line L7 (-14.5654, -10.3029) -> (233.4346, -10.3029)
  arc A7 (233.4346, -10.3029) -> (234.4346, -9.3029) centre (233.4346, -9.3029) ccw
  point P0 (0, 0)
  dimension "d97" = 2
  constraints: 8 end point, 8 point on circle, 4 centre point, 7 other
  measures "d97" radial gap between concentric circles of A3 A7
extrude "Extrusion3" add sketch "Skizze3" along normal blind 6.25
fillet "Rundung1" radius 1 8 edges at (16.6867, -11.4242, -6.25) (-109.4346, -12.3029, -6.25) (-235.5559, -11.4242, -6.25) (-236.4346, 28.6971, -6.25) (-235.5559, 68.8184, -6.25) (-109.4346, 69.6971, -6.25) (16.6867, 68.8184, -6.25) (17.5654, 28.6971, -6.25)
sketch "Skizze4" plane through (0, 0, 1.5) normal (0, 0, 1) x (1, 0, 0)
  circle A0 centre (-230.6946, -6.6429) radius 1.6
  circle A1 centre (-230.7946, 30.6571) radius 1.6
  circle A2 centre (-176.2946, 60.4571) radius 1.6
  circle A3 centre (-121.1946, 0.9571) radius 1.6
  circle A4 centre (-100.1946, 48.7571) radius 1.6
  circle A5 centre (11.9054, -6.6429) radius 1.6
  circle A6 centre (12.1054, 46.6571) radius 1.6
  circle A7 centre (-230.6946, -6.6429) radius 2.25
  circle A8 centre (-230.7946, 30.6571) radius 2.25
  circle A9 centre (-176.2946, 60.4571) radius 2.25
  circle A10 centre (-121.1946, 0.9571) radius 2.25
  circle A11 centre (-100.1946, 48.7571) radius 2.25
  circle A12 centre (11.9054, -6.6429) radius 2.25
  circle A13 centre (12.1054, 46.6571) radius 2.25
  point P0 (0, 0)
extrude "Extrusion4" add sketch "Skizze4" along normal blind 3.66 contours A0 | A1 | A3 | A4 | A5 | A6 | A7 | A8 | A10 | A11 | A12 | A13
hole "Bohrung1" at (-230.7946, 30.6571, 5.16) at (-230.6946, -6.6429, 5.16) at (-121.1946, 0.9571, 5.16) at (-100.1946, 48.7571, 5.16) at (12.1054, 46.6571, 5.16) at (11.9054, -6.6429, 5.16) direction (0, 0, -1) diameter 2.459 depth 3.66 tip angle 118 thread size "M3x0.5" class "6H" standard "ANSI Metric M Profile"
fillet "Rundung2" radius 2 6 edges at (-102.4446, 48.7571, 1.5) (9.8554, 46.6571, 1.5) (9.6554, -6.6429, 1.5) (-123.4446, 0.9571, 1.5) (-232.9446, -6.6429, 1.5) (-233.0446, 30.6571, 1.5)
sketch "Skizze6" plane through (-233.4346, 68.1971, 1.5) normal (0, -1, 0) x (1, 0, 0)
  line L0 (10.65, 5.1375) -> (10.05, 5.1375) projected
  line L1 (2.01, 5.1375) -> (1.41, 5.1375) projected
  line L2 (1.41, 6.6375) -> (10.65, 6.6375) construction
  line L3 (1.41, 5.1375) -> (10.65, 5.1375)
  line L4 (10.65, 8.1375) -> (1.41, 8.1375)
  arc A0 (1.41, 8.1375) -> (1.41, 5.1375) centre (1.41, 6.6375) ccw
  arc A1 (10.65, 5.1375) -> (10.65, 8.1375) centre (10.65, 6.6375) ccw
  point P0 (233.4346, -1.5)
  point P1 (6.03, 6.6375)
  dimension "d118" = 3
  constraints: 8 end point, 4 point on circle, 4 tangent, 3 coincident, 2 centre point, 1 horizontal, 1 midpoint, 1 parallel
  measures "d118" diameter of A1
extrude "Extrusion5" cut sketch "Skizze6" against normal through all
